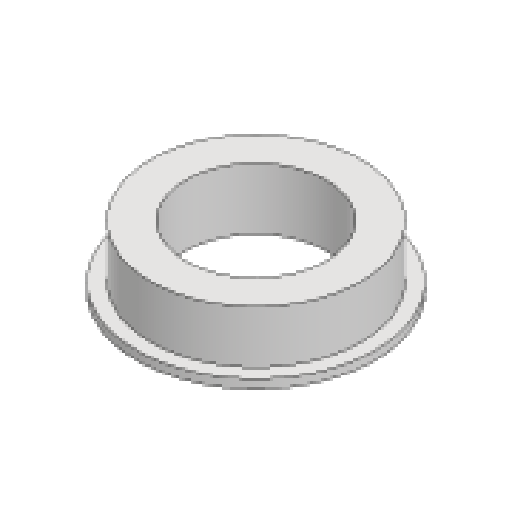
# Autodesk Inventor part: 8x12x3.5 flanged bearing
Saved by Autodesk Inventor 2023 (Build 270158000, 158)
## iProperties
Created: 2022-10-29
Part Number: 8x12x3.5 flanged bearing
Material: Generic
Document SubType Name: Modeling
Designer: deli
Density: 1 g/cm^3
Appearance: Default
Author: deli
Autodesk Inventor part; units mm, degrees
ref_plane "YZ Plane" through (0, 0, 0) normal (1, 0, 0) x (0, 1, 0)
ref_plane "XZ Plane" through (0, 0, 0) normal (0, 1, 0) x (-1, 0, 0)
ref_plane "XY Plane" through (0, 0, 0) normal (0, 0, 1) x (1, 0, 0)
sketch "Sketch1" plane through (0, 0, 0) normal (0, 1, 0) x (-1, 0, 0)
  circle A0 centre (8.6225, 15.3447) radius 4
  circle A1 centre (8.6225, 15.3447) radius 6.8
  point P0 (0, 0)
  dimension "d0" = 8
  dimension "d1" = 13.6
  constraints: 2 centre point, 1 coincident
  measures "d0" diameter of A0
  measures "d1" diameter of A1
extrude "Extrusion1" add sketch "Sketch1" along normal blind 3.5
sketch "Sketch2" plane through (-8.6225, 3.5, 15.3447) normal (0, 1, 0) x (1, 0, 0)
  circle A0 centre (0, 0) radius 6.8 projected
  circle A1 centre (0, 0) radius 6
  point P0 (8.6225, 15.3447)
  dimension "d4" = 12
  constraints: 1 centre point, 1 coincident
  measures "d4" diameter of A1
extrude "Extrusion2" cut sketch "Sketch2" against normal blind 3
body "Solid1"
